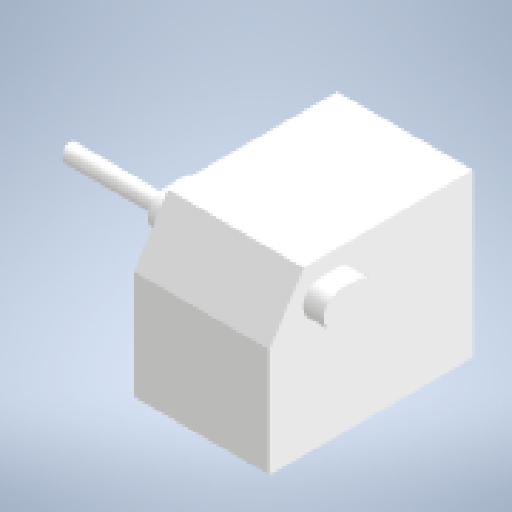
# Autodesk Inventor part: Motor
Saved by Autodesk Inventor 2024.1 (Build 281209000, 209)
## iProperties
Created: 2024-07-01
Part Number: Motor
Material: 一般
Document SubType Name: Modeling
Designer: hibik
Density: 1 g/cm^3
Appearance: 既定
Author: hibik
Autodesk Inventor part; units mm, degrees
ref_plane "YZ Plane" through (0, 0, 0) normal (1, 0, 0) x (0, 1, 0)
ref_plane "XZ Plane" through (0, 0, 0) normal (0, 1, 0) x (-1, 0, 0)
sketch "スケッチ1" plane through (0, 0, 0) normal (0, 1, 0) x (-1, 0, 0)
  line L0 (0, 0) -> (20, 0)
  line L1 (20, 0) -> (20, -30)
  line L2 (20, -30) -> (0, -30)
  line L3 (0, -30) -> (0, 0)
  dimension "d0" = 20
  dimension "d1" = 30
  constraints: 8 end point, 2 parallel, 1 horizontal, 1 perpendicular
  measures "d0" distance of L1.end L2.end
  measures "d1" distance of L0.end L1.end
extrude "押し出し1" add sketch "スケッチ1" along normal blind 24
sketch "スケッチ2" plane through (0, 0, 0) normal (1, 0, 0) x (0, 0, -1)
  line L0 (0, 0) -> (0, 24) projected
  line L1 (0, 16) -> (0, 24)
  line L2 (0, 24) -> (5, 24)
  line L3 (5, 24) -> (0, 16)
  dimension "d4" = 5
  dimension "d5" = 8
  constraints: 6 end point, 1 collinear, 1 perpendicular, 1 point on line
  measures "d4" distance of L0.end L2.end
  measures "d5" distance from line of L2 L1.start
extrude "押し出し2" cut sketch "スケッチ2" against normal through all
sketch "スケッチ3" plane through (-20, 0, -30) normal (-1, 0, 0) x (0, 0, 1)
  circle A0 centre (22.5, 19) radius 2.5
  line L0 (30, 0) -> (30, 16) projected
  line L1 (0, 24) -> (25, 24) projected
  circle A1 centre (20, 19) radius 2.5
  line L2 (17.5, 21.5) -> (25, 21.5)
  line L3 (25, 21.5) -> (25, 16.5) construction
  line L4 (25, 16.5) -> (17.5, 16.5)
  line L5 (17.5, 16.5) -> (17.5, 21.5) construction
  point P0 (22.5, 21.5)
  point P1 (20, 21.5)
  point P2 (20, 16.5)
  point P3 (22.5, 16.5)
  dimension "d8" = 5
  dimension "d9" = 7.5
  dimension "d10" = 5
  dimension "d11" = 5
  dimension "d12" = 7.5
  constraints: 8 end point, 4 tangent, 2 centre point, 2 parallel, 1 horizontal, 1 horizontal alignment, 1 perpendicular
  measures "d8" diameter of A0
  measures "d9" distance from line of L0 A0.centre
  measures "d10" distance from line of L1 A0.centre
  measures "d11" diameter of A1
  measures "d12" distance of L2.start L2.end
extrude "押し出し3" add sketch "スケッチ3" along normal blind 3
ref_plane "作業平面1" through (-10, 0, -30) normal (-1, 0, 0) x (0, 0, 1)
mirror "ミラー1" about plane through (-10, 0, -30) normal (-1, 0, 0) of "押し出し3"
sketch "スケッチ4" plane through (3, 19, -10) normal (1, 0, 0) x (0, 0, -1)
  arc A0 (-2.5, 2.5) -> (-2.5, -2.5) centre (-2.5, 0) ccw projected
  circle A1 centre (-2.5, 0) radius 1.25
  point P0 (-10, -19)
  dimension "d16" = 2.5
  constraints: 1 centre point, 1 coincident
  measures "d16" diameter of A1
extrude "押し出し4" add sketch "スケッチ4" against normal blind 50
